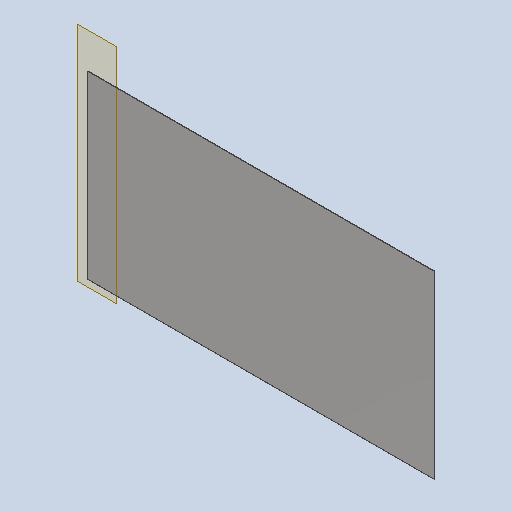
# Autodesk Inventor part: GEAR_REST
Saved by Autodesk Inventor 2024 (Build 280153000, 153)
## iProperties
Created: 2024-04-16
Part Number: GEAR_REST
Material: Stainless Steel
Document SubType Name: Sheet Metal
Designer: teeta
Density: 8 g/cm^3
Sheet Metal Rule: Default_mm
Appearance: Semi-Polished
Author: teeta
Autodesk Inventor part; units mm, degrees
ref_plane "YZ Plane" through (0, 0, 0) normal (1, 0, 0) x (0, 1, 0)
ref_plane "XZ Plane" through (0, 0, 0) normal (0, 1, 0) x (-1, 0, 0)
ref_plane "XY Plane" through (0, 0, 0) normal (0, 0, 1) x (1, 0, 0)
ref_plane "Work Plane1" through (-355.55, 0, 0) normal (0, 0, 1) x (1, 0, 0)
sketch "Sketch1" plane through (-355.55, 0, 0) normal (0, 0, 1) x (1, 0, 0)
  line L0 (-28.775, -3.175) -> (346.225, -3.175)
  line L1 (346.225, -3.175) -> (346.225, 191.825)
  line L2 (346.225, 191.825) -> (-28.775, 191.825)
  line L3 (-28.775, 191.825) -> (-28.775, -3.175)
  line L4 (539.675, -3.175) -> (-222.225, -3.175)
  line L5 (-44.45, 0) -> (-44.45, 174.6)
  line L6 (361.9, 0) -> (361.9, 174.6)
  point P0 (355.55, 0)
  dimension "d0" = 195
  dimension "d1" = 375
  dimension "d2" = 15.675
  dimension "d3" = 15.675
  measures "d0" distance of L2.end L0.start
  measures "d1" distance of L1.end L2.end
  measures "d2" distance between parallel lines of L1 L6
  measures "d3" distance between parallel lines of L3 L5
extrude "Plate1" add sketch "Sketch1" along normal blind 0.5
equation "\"d4\" = Thickness"
equation "\"BendRadius\" = Thickness"
equation "\"BendReliefWidth\" = Thickness"
equation "\"BendReliefDepth\" = 0.5 * Thickness"
equation "\"CornerReliefSize\" = 4 * Thickness"
equation "\"MinimumRemnant\" = 2 * Thickness"
equation "\"TransitionRadius\" = BendRadius"
equation "\"JacobiRadiusSize\" = BendRadius"
equation "\"GapSize\" = Thickness"
equation "\"Thickness\" = 0.5"
body "Solid1"
